Autodesk Fusion 360 part; units mm, degrees
(part 2 of 3)
  line L328 (-114.4464, -236.9799) -> (-114.4464, -230.9799)
  line L329 (-114.4464, -230.9799) -> (-108.4464, -230.9799)
  line L330 (-108.4464, -230.9799) -> (-108.4464, -236.9799)
  line L331 (-108.4464, -236.9799) -> (-114.4464, -236.9799)
  line L332 (53.6667, -182.5) -> (47.6667, -182.5)
  line L333 (47.6667, -182.5) -> (47.6667, -176.5)
  line L334 (47.6667, -176.5) -> (53.6667, -176.5)
  line L335 (53.6667, -176.5) -> (53.6667, -182.5)
  line L336 (61.3333, -182.5) -> (55.3333, -182.5)
  line L337 (55.3333, -182.5) -> (55.3333, -176.5)
  line L338 (55.3333, -176.5) -> (61.3333, -176.5)
  line L339 (61.3333, -176.5) -> (61.3333, -182.5)
  line L340 (69, -182.5) -> (63, -182.5)
  line L341 (63, -182.5) -> (63, -176.5)
  line L342 (63, -176.5) -> (69, -176.5)
  line L343 (69, -176.5) -> (69, -182.5)
  line L344 (76.6667, -182.5) -> (70.6667, -182.5)
  line L345 (70.6667, -182.5) -> (70.6667, -176.5)
  line L346 (70.6667, -176.5) -> (76.6667, -176.5)
  line L347 (76.6667, -176.5) -> (76.6667, -182.5)
  line L348 (84.3333, -182.5) -> (78.3333, -182.5)
  line L349 (78.3333, -182.5) -> (78.3333, -176.5)
  line L350 (78.3333, -176.5) -> (84.3333, -176.5)
  line L351 (84.3333, -176.5) -> (84.3333, -182.5)
  line L352 (92, -182.5) -> (86, -182.5)
  line L353 (86, -182.5) -> (86, -176.5)
  line L354 (86, -176.5) -> (92, -176.5)
  line L355 (92, -176.5) -> (92, -182.5)
  line L356 (99.6667, -182.5) -> (93.6667, -182.5)
  line L357 (93.6667, -182.5) -> (93.6667, -176.5)
  line L358 (93.6667, -176.5) -> (99.6667, -176.5)
  line L359 (99.6667, -176.5) -> (99.6667, -182.5)
  line L360 (107.3333, -182.5) -> (101.3333, -182.5)
  line L361 (101.3333, -182.5) -> (101.3333, -176.5)
  line L362 (101.3333, -176.5) -> (107.3333, -176.5)
  line L363 (107.3333, -176.5) -> (107.3333, -182.5)
  line L364 (53.6667, -190.3571) -> (47.6667, -190.3571)
  line L365 (47.6667, -190.3571) -> (47.6667, -184.3571)
  line L366 (47.6667, -184.3571) -> (53.6667, -184.3571)
  line L367 (53.6667, -184.3571) -> (53.6667, -190.3571)
  line L368 (61.3333, -190.3571) -> (55.3333, -190.3571)
  line L369 (55.3333, -190.3571) -> (55.3333, -184.3571)
  line L370 (55.3333, -184.3571) -> (61.3333, -184.3571)
  line L371 (61.3333, -184.3571) -> (61.3333, -190.3571)
  line L372 (69, -190.3571) -> (63, -190.3571)
  line L373 (63, -190.3571) -> (63, -184.3571)
  line L374 (63, -184.3571) -> (69, -184.3571)
  line L375 (69, -184.3571) -> (69, -190.3571)
  line L376 (76.6667, -190.3571) -> (70.6667, -190.3571)
  line L377 (70.6667, -190.3571) -> (70.6667, -184.3571)
  line L378 (70.6667, -184.3571) -> (76.6667, -184.3571)
  line L379 (76.6667, -184.3571) -> (76.6667, -190.3571)
  line L380 (84.3333, -190.3571) -> (78.3333, -190.3571)
  line L381 (78.3333, -190.3571) -> (78.3333, -184.3571)
  line L382 (78.3333, -184.3571) -> (84.3333, -184.3571)
  line L383 (84.3333, -184.3571) -> (84.3333, -190.3571)
  line L384 (92, -190.3571) -> (86, -190.3571)
  line L385 (86, -190.3571) -> (86, -184.3571)
  line L386 (86, -184.3571) -> (92, -184.3571)
  line L387 (92, -184.3571) -> (92, -190.3571)
  line L388 (99.6667, -190.3571) -> (93.6667, -190.3571)
  line L389 (93.6667, -190.3571) -> (93.6667, -184.3571)
  line L390 (93.6667, -184.3571) -> (99.6667, -184.3571)
  line L391 (99.6667, -184.3571) -> (99.6667, -190.3571)
  line L392 (107.3333, -190.3571) -> (101.3333, -190.3571)
  line L393 (101.3333, -190.3571) -> (101.3333, -184.3571)
  line L394 (101.3333, -184.3571) -> (107.3333, -184.3571)
  line L395 (107.3333, -184.3571) -> (107.3333, -190.3571)
  line L396 (53.6667, -198.2143) -> (47.6667, -198.2143)
  line L397 (47.6667, -198.2143) -> (47.6667, -192.2143)
  line L398 (47.6667, -192.2143) -> (53.6667, -192.2143)
  line L399 (53.6667, -192.2143) -> (53.6667, -198.2143)
  line L400 (61.3333, -198.2143) -> (55.3333, -198.2143)
  line L401 (55.3333, -198.2143) -> (55.3333, -192.2143)
  line L402 (55.3333, -192.2143) -> (61.3333, -192.2143)
  line L403 (61.3333, -192.2143) -> (61.3333, -198.2143)
  line L404 (69, -198.2143) -> (63, -198.2143)
  line L405 (63, -198.2143) -> (63, -192.2143)
  line L406 (63, -192.2143) -> (69, -192.2143)
  line L407 (69, -192.2143) -> (69, -198.2143)
  line L408 (76.6667, -198.2143) -> (70.6667, -198.2143)
  line L409 (70.6667, -198.2143) -> (70.6667, -192.2143)
  line L410 (70.6667, -192.2143) -> (76.6667, -192.2143)
  line L411 (76.6667, -192.2143) -> (76.6667, -198.2143)
  line L412 (84.3333, -198.2143) -> (78.3333, -198.2143)
  line L413 (78.3333, -198.2143) -> (78.3333, -192.2143)
  line L414 (78.3333, -192.2143) -> (84.3333, -192.2143)
  line L415 (84.3333, -192.2143) -> (84.3333, -198.2143)
  line L416 (92, -198.2143) -> (86, -198.2143)
  line L417 (86, -198.2143) -> (86, -192.2143)
  line L418 (86, -192.2143) -> (92, -192.2143)
  line L419 (92, -192.2143) -> (92, -198.2143)
  line L420 (99.6667, -198.2143) -> (93.6667, -198.2143)
  line L421 (93.6667, -198.2143) -> (93.6667, -192.2143)
  line L422 (93.6667, -192.2143) -> (99.6667, -192.2143)
  line L423 (99.6667, -192.2143) -> (99.6667, -198.2143)
  line L424 (107.3333, -198.2143) -> (101.3333, -198.2143)
  line L425 (101.3333, -198.2143) -> (101.3333, -192.2143)
  line L426 (101.3333, -192.2143) -> (107.3333, -192.2143)
  line L427 (107.3333, -192.2143) -> (107.3333, -198.2143)
  line L428 (53.6667, -206.0714) -> (47.6667, -206.0714)
  line L429 (47.6667, -206.0714) -> (47.6667, -200.0714)
  line L430 (47.6667, -200.0714) -> (53.6667, -200.0714)
  line L431 (53.6667, -200.0714) -> (53.6667, -206.0714)
  line L432 (61.3333, -206.0714) -> (55.3333, -206.0714)
  line L433 (55.3333, -206.0714) -> (55.3333, -200.0714)
  line L434 (55.3333, -200.0714) -> (61.3333, -200.0714)
  line L435 (61.3333, -200.0714) -> (61.3333, -206.0714)
  line L436 (69, -206.0714) -> (63, -206.0714)
  line L437 (63, -206.0714) -> (63, -200.0714)
  line L438 (63, -200.0714) -> (69, -200.0714)
  line L439 (69, -200.0714) -> (69, -206.0714)
  line L440 (76.6667, -206.0714) -> (70.6667, -206.0714)
  line L441 (70.6667, -206.0714) -> (70.6667, -200.0714)
  line L442 (70.6667, -200.0714) -> (76.6667, -200.0714)
  line L443 (76.6667, -200.0714) -> (76.6667, -206.0714)
  line L444 (84.3333, -206.0714) -> (78.3333, -206.0714)
  line L445 (78.3333, -206.0714) -> (78.3333, -200.0714)
  line L446 (78.3333, -200.0714) -> (84.3333, -200.0714)
  line L447 (84.3333, -200.0714) -> (84.3333, -206.0714)
  line L448 (92, -206.0714) -> (86, -206.0714)
  line L449 (86, -206.0714) -> (86, -200.0714)
  line L450 (86, -200.0714) -> (92, -200.0714)
  line L451 (92, -200.0714) -> (92, -206.0714)
  line L452 (99.6667, -206.0714) -> (93.6667, -206.0714)
  line L453 (93.6667, -206.0714) -> (93.6667, -200.0714)
  line L454 (93.6667, -200.0714) -> (99.6667, -200.0714)
  line L455 (99.6667, -200.0714) -> (99.6667, -206.0714)
  line L456 (107.3333, -206.0714) -> (101.3333, -206.0714)
  line L457 (101.3333, -206.0714) -> (101.3333, -200.0714)
  line L458 (101.3333, -200.0714) -> (107.3333, -200.0714)
  line L459 (107.3333, -200.0714) -> (107.3333, -206.0714)
  line L460 (53.6667, -213.9286) -> (47.6667, -213.9286)
  line L461 (47.6667, -213.9286) -> (47.6667, -207.9286)
  line L462 (47.6667, -207.9286) -> (53.6667, -207.9286)
  line L463 (53.6667, -207.9286) -> (53.6667, -213.9286)
  line L464 (61.3333, -213.9286) -> (55.3333, -213.9286)
  line L465 (55.3333, -213.9286) -> (55.3333, -207.9286)
  line L466 (55.3333, -207.9286) -> (61.3333, -207.9286)
  line L467 (61.3333, -207.9286) -> (61.3333, -213.9286)
  line L468 (69, -213.9286) -> (63, -213.9286)
  line L469 (63, -213.9286) -> (63, -207.9286)
  line L470 (63, -207.9286) -> (69, -207.9286)
  line L471 (69, -207.9286) -> (69, -213.9286)
  line L472 (76.6667, -213.9286) -> (70.6667, -213.9286)
  line L473 (70.6667, -213.9286) -> (70.6667, -207.9286)
  line L474 (70.6667, -207.9286) -> (76.6667, -207.9286)
  line L475 (76.6667, -207.9286) -> (76.6667, -213.9286)
  line L476 (84.3333, -213.9286) -> (78.3333, -213.9286)
  line L477 (78.3333, -213.9286) -> (78.3333, -207.9286)
  line L478 (78.3333, -207.9286) -> (84.3333, -207.9286)
  line L479 (84.3333, -207.9286) -> (84.3333, -213.9286)
  line L480 (92, -213.9286) -> (86, -213.9286)
  line L481 (86, -213.9286) -> (86, -207.9286)
  line L482 (86, -207.9286) -> (92, -207.9286)
  line L483 (92, -207.9286) -> (92, -213.9286)
  line L484 (99.6667, -213.9286) -> (93.6667, -213.9286)
  line L485 (93.6667, -213.9286) -> (93.6667, -207.9286)
  line L486 (93.6667, -207.9286) -> (99.6667, -207.9286)
  line L487 (99.6667, -207.9286) -> (99.6667, -213.9286)
  line L488 (107.3333, -213.9286) -> (101.3333, -213.9286)
  line L489 (101.3333, -213.9286) -> (101.3333, -207.9286)
  line L490 (101.3333, -207.9286) -> (107.3333, -207.9286)
  line L491 (107.3333, -207.9286) -> (107.3333, -213.9286)
  line L492 (53.6667, -221.7857) -> (47.6667, -221.7857)
  line L493 (47.6667, -221.7857) -> (47.6667, -215.7857)
  line L494 (47.6667, -215.7857) -> (53.6667, -215.7857)
  line L495 (53.6667, -215.7857) -> (53.6667, -221.7857)
  line L496 (61.3333, -221.7857) -> (55.3333, -221.7857)
  line L497 (55.3333, -221.7857) -> (55.3333, -215.7857)
  line L498 (55.3333, -215.7857) -> (61.3333, -215.7857)
  line L499 (61.3333, -215.7857) -> (61.3333, -221.7857)
  line L500 (69, -221.7857) -> (63, -221.7857)
  line L501 (63, -221.7857) -> (63, -215.7857)
  line L502 (63, -215.7857) -> (69, -215.7857)
  line L503 (69, -215.7857) -> (69, -221.7857)
  line L504 (76.6667, -221.7857) -> (70.6667, -221.7857)
  line L505 (70.6667, -221.7857) -> (70.6667, -215.7857)
  line L506 (70.6667, -215.7857) -> (76.6667, -215.7857)
  line L507 (76.6667, -215.7857) -> (76.6667, -221.7857)
  line L508 (84.3333, -221.7857) -> (78.3333, -221.7857)
  line L509 (78.3333, -221.7857) -> (78.3333, -215.7857)
  line L510 (78.3333, -215.7857) -> (84.3333, -215.7857)
  line L511 (84.3333, -215.7857) -> (84.3333, -221.7857)
  line L512 (92, -221.7857) -> (86, -221.7857)
  line L513 (86, -221.7857) -> (86, -215.7857)
  line L514 (86, -215.7857) -> (92, -215.7857)
  line L515 (92, -215.7857) -> (92, -221.7857)
  line L516 (99.6667, -221.7857) -> (93.6667, -221.7857)
  line L517 (93.6667, -221.7857) -> (93.6667, -215.7857)
  line L518 (93.6667, -215.7857) -> (99.6667, -215.7857)
  line L519 (99.6667, -215.7857) -> (99.6667, -221.7857)
  line L520 (107.3333, -221.7857) -> (101.3333, -221.7857)
  line L521 (101.3333, -221.7857) -> (101.3333, -215.7857)
  line L522 (101.3333, -215.7857) -> (107.3333, -215.7857)
  line L523 (107.3333, -215.7857) -> (107.3333, -221.7857)
  line L524 (53.6667, -229.6429) -> (47.6667, -229.6429)
  line L525 (47.6667, -229.6429) -> (47.6667, -223.6429)
  line L526 (47.6667, -223.6429) -> (53.6667, -223.6429)
  line L527 (53.6667, -223.6429) -> (53.6667, -229.6429)
  line L528 (61.3333, -229.6429) -> (55.3333, -229.6429)
  line L529 (55.3333, -229.6429) -> (55.3333, -223.6429)
  line L530 (55.3333, -223.6429) -> (61.3333, -223.6429)
  line L531 (61.3333, -223.6429) -> (61.3333, -229.6429)
  line L532 (69, -229.6429) -> (63, -229.6429)
  line L533 (63, -229.6429) -> (63, -223.6429)
  line L534 (63, -223.6429) -> (69, -223.6429)
  line L535 (69, -223.6429) -> (69, -229.6429)
  line L536 (76.6667, -229.6429) -> (70.6667, -229.6429)
  line L537 (70.6667, -229.6429) -> (70.6667, -223.6429)
  line L538 (70.6667, -223.6429) -> (76.6667, -223.6429)
  line L539 (76.6667, -223.6429) -> (76.6667, -229.6429)
  line L540 (84.3333, -229.6429) -> (78.3333, -229.6429)
  line L541 (78.3333, -229.6429) -> (78.3333, -223.6429)
  line L542 (78.3333, -223.6429) -> (84.3333, -223.6429)
  line L543 (84.3333, -223.6429) -> (84.3333, -229.6429)
  line L544 (92, -229.6429) -> (86, -229.6429)
  line L545 (86, -229.6429) -> (86, -223.6429)
  line L546 (86, -223.6429) -> (92, -223.6429)
  line L547 (92, -223.6429) -> (92, -229.6429)
  line L548 (99.6667, -229.6429) -> (93.6667, -229.6429)
  line L549 (93.6667, -229.6429) -> (93.6667, -223.6429)
  line L550 (93.6667, -223.6429) -> (99.6667, -223.6429)
  line L551 (99.6667, -223.6429) -> (99.6667, -229.6429)
  line L552 (107.3333, -229.6429) -> (101.3333, -229.6429)
  line L553 (101.3333, -229.6429) -> (101.3333, -223.6429)
  line L554 (101.3333, -223.6429) -> (107.3333, -223.6429)
  line L555 (107.3333, -223.6429) -> (107.3333, -229.6429)
  line L556 (53.6667, -237.5) -> (47.6667, -237.5)
  line L557 (47.6667, -237.5) -> (47.6667, -231.5)
  line L558 (47.6667, -231.5) -> (53.6667, -231.5)
  line L559 (53.6667, -231.5) -> (53.6667, -237.5)
  line L560 (61.3333, -237.5) -> (55.3333, -237.5)
  line L561 (55.3333, -237.5) -> (55.3333, -231.5)
  line L562 (55.3333, -231.5) -> (61.3333, -231.5)
  line L563 (61.3333, -231.5) -> (61.3333, -237.5)
  line L564 (69, -237.5) -> (63, -237.5)
  line L565 (63, -237.5) -> (63, -231.5)
  line L566 (63, -231.5) -> (69, -231.5)
  line L567 (69, -231.5) -> (69, -237.5)
  line L568 (76.6667, -237.5) -> (70.6667, -237.5)
  line L569 (70.6667, -237.5) -> (70.6667, -231.5)
  line L570 (70.6667, -231.5) -> (76.6667, -231.5)
  line L571 (76.6667, -231.5) -> (76.6667, -237.5)
  line L572 (84.3333, -237.5) -> (78.3333, -237.5)
  line L573 (78.3333, -237.5) -> (78.3333, -231.5)
  line L574 (78.3333, -231.5) -> (84.3333, -231.5)
  line L575 (84.3333, -231.5) -> (84.3333, -237.5)
  line L576 (92, -237.5) -> (86, -237.5)
  line L577 (86, -237.5) -> (86, -231.5)
  line L578 (86, -231.5) -> (92, -231.5)
  line L579 (92, -231.5) -> (92, -237.5)
  line L580 (99.6667, -237.5) -> (93.6667, -237.5)
  line L581 (93.6667, -237.5) -> (93.6667, -231.5)
  line L582 (93.6667, -231.5) -> (99.6667, -231.5)
  line L583 (99.6667, -231.5) -> (99.6667, -237.5)
  line L584 (101.3333, -231.5) -> (107.3333, -231.5)
  line L585 (107.3333, -231.5) -> (107.3333, -237.5)
  line L586 (107.3333, -237.5) -> (101.3333, -237.5)
  line L587 (101.3333, -237.5) -> (101.3333, -231.5)
  line L588 (156, -177) -> (156, -160)
  line L589 (156, -160) -> (143.1111, -160)
  line L590 (143.1111, -160) -> (143.1111, -155)
  line L591 (143.1111, -155) -> (125.2222, -155)
  line L592 (125.2222, -155) -> (125.2222, -160)
  line L593 (125.2222, -160) -> (107.3333, -160)
  line L594 (107.3333, -160) -> (107.3333, -155)
  line L595 (107.3333, -155) -> (89.4444, -155)
  line L596 (89.4444, -155) -> (89.4444, -160)
  line L597 (89.4444, -160) -> (71.5556, -160)
  line L598 (71.5556, -160) -> (71.5556, -155)
  line L599 (71.5556, -155) -> (53.6667, -155)
  line L600 (53.6667, -155) -> (53.6667, -160)
  line L601 (53.6667, -160) -> (35.7778, -160)
  line L602 (35.7778, -160) -> (35.7778, -155)
  line L603 (35.7778, -155) -> (17.8889, -155)
  line L604 (17.8889, -155) -> (17.8889, -160)
  line L605 (17.8889, -160) -> (5, -160)
  line L606 (5, -160) -> (5, -177)
  line L607 (5, -177) -> (0, -177)
  line L608 (0, -177) -> (0, -199)
  line L609 (0, -199) -> (5, -199)
  line L610 (5, -199) -> (5, -221)
  line L611 (5, -221) -> (0, -221)
  line L612 (0, -221) -> (0, -243)
  line L613 (0, -243) -> (5, -243)
  line L614 (5, -243) -> (5, -265)
  line L615 (5, -265) -> (156, -265)
  line L616 (156, -265) -> (156, -243)
  line L617 (156, -243) -> (161, -243)
  line L618 (161, -243) -> (161, -221)
  line L619 (161, -221) -> (156, -221)
  line L620 (156, -221) -> (156, -199)
  line L621 (156, -199) -> (161, -199)
  line L622 (161, -199) -> (161, -177)
  line L623 (161, -177) -> (156, -177)
  line L624 (264.348, -187.6487) -> (264.348, -172.6487)
  line L625 (264.348, -172.6487) -> (270.348, -172.6487)
  line L626 (270.348, -172.6487) -> (270.348, -187.6487)
  line L627 (270.348, -187.6487) -> (264.348, -187.6487)
  line L628 (256.0147, -187.6487) -> (256.0147, -172.6487)
  line L629 (256.0147, -172.6487) -> (262.0147, -172.6487)
  line L630 (262.0147, -172.6487) -> (262.0147, -187.6487)
  line L631 (262.0147, -187.6487) -> (256.0147, -187.6487)
  line L632 (247.6814, -187.6487) -> (247.6814, -172.6487)
  line L633 (247.6814, -172.6487) -> (253.6814, -172.6487)
  line L634 (253.6814, -172.6487) -> (253.6814, -187.6487)
  line L635 (253.6814, -187.6487) -> (247.6814, -187.6487)
  line L636 (239.348, -187.6487) -> (239.348, -172.6487)
  line L637 (239.348, -172.6487) -> (245.348, -172.6487)
  line L638 (245.348, -172.6487) -> (245.348, -187.6487)
  line L639 (245.348, -187.6487) -> (239.348, -187.6487)
  line L640 (231.0147, -187.6487) -> (231.0147, -172.6487)
  line L641 (231.0147, -172.6487) -> (237.0147, -172.6487)
  line L642 (237.0147, -172.6487) -> (237.0147, -187.6487)
  line L643 (237.0147, -187.6487) -> (231.0147, -187.6487)
  line L644 (222.6814, -187.6487) -> (222.6814, -172.6487)
  line L645 (222.6814, -172.6487) -> (228.6814, -172.6487)
  line L646 (228.6814, -172.6487) -> (228.6814, -187.6487)
  line L647 (228.6814, -187.6487) -> (222.6814, -187.6487)
  line L648 (214.348, -187.6487) -> (214.348, -172.6487)
  line L649 (214.348, -172.6487) -> (220.348, -172.6487)
  line L650 (220.348, -172.6487) -> (220.348, -187.6487)
  line L651 (220.348, -187.6487) -> (214.348, -187.6487)
  line L652 (206.0147, -187.6487) -> (206.0147, -172.6487)
  line L653 (206.0147, -172.6487) -> (212.0147, -172.6487)
  line L654 (212.0147, -172.6487) -> (212.0147, -187.6487)
  line L655 (212.0147, -187.6487) -> (206.0147, -187.6487)
  line L656 (197.6814, -187.6487) -> (197.6814, -172.6487)
  line L657 (197.6814, -172.6487) -> (203.6814, -172.6487)
  line L658 (203.6814, -172.6487) -> (203.6814, -187.6487)
  line L659 (203.6814, -187.6487) -> (197.6814, -187.6487)
  line L660 (189.348, -187.6487) -> (189.348, -172.6487)
  line L661 (189.348, -172.6487) -> (195.348, -172.6487)
  line L662 (195.348, -172.6487) -> (195.348, -187.6487)
  line L663 (195.348, -187.6487) -> (189.348, -187.6487)
  line L664 (309.348, -176.3154) -> (314.348, -176.3154)
  line L665 (314.348, -176.3154) -> (314.348, -159.3154)
  line L666 (314.348, -159.3154) -> (300.7117, -159.3154)
  line L667 (300.7117, -159.3154) -> (300.7117, -154.3154)
  line L668 (300.7117, -154.3154) -> (287.0753, -154.3154)
  line L669 (287.0753, -154.3154) -> (287.0753, -159.3154)
  line L670 (287.0753, -159.3154) -> (273.4389, -159.3154)
  line L671 (273.4389, -159.3154) -> (273.4389, -154.3154)
  line L672 (273.4389, -154.3154) -> (259.8026, -154.3154)
  line L673 (259.8026, -154.3154) -> (259.8026, -159.3154)
  line L674 (259.8026, -159.3154) -> (246.1662, -159.3154)
  line L675 (246.1662, -159.3154) -> (246.1662, -154.3154)
  line L676 (246.1662, -154.3154) -> (232.5298, -154.3154)
  line L677 (232.5298, -154.3154) -> (232.5298, -159.3154)
  line L678 (232.5298, -159.3154) -> (218.8935, -159.3154)
  line L679 (218.8935, -159.3154) -> (218.8935, -154.3154)
  line L680 (218.8935, -154.3154) -> (205.2571, -154.3154)
  line L681 (205.2571, -154.3154) -> (205.2571, -159.3154)
  line L682 (205.2571, -159.3154) -> (191.6208, -159.3154)
  line L683 (191.6208, -159.3154) -> (191.6208, -154.3154)
  line L684 (191.6208, -154.3154) -> (177.9844, -154.3154)
  line L685 (177.9844, -154.3154) -> (177.9844, -159.3154)
  line L686 (177.9844, -159.3154) -> (164.348, -159.3154)
  line L687 (164.348, -159.3154) -> (164.348, -176.3154)
  line L688 (164.348, -176.3154) -> (169.348, -176.3154)
  line L689 (169.348, -176.3154) -> (169.348, -198.3154)
  line L690 (169.348, -198.3154) -> (164.348, -198.3154)
  line L691 (164.348, -198.3154) -> (164.348, -220.3154)
  line L692 (164.348, -220.3154) -> (169.348, -220.3154)
  line L693 (169.348, -220.3154) -> (169.348, -242.3154)
  line L694 (169.348, -242.3154) -> (164.348, -242.3154)
  line L695 (164.348, -242.3154) -> (164.348, -264.3154)
  line L696 (164.348, -264.3154) -> (314.348, -264.3154)
  line L697 (314.348, -264.3154) -> (314.348, -242.3154)
  line L698 (314.348, -242.3154) -> (309.348, -242.3154)
  line L699 (309.348, -242.3154) -> (309.348, -220.3154)
  line L700 (309.348, -220.3154) -> (314.348, -220.3154)
  line L701 (314.348, -220.3154) -> (314.348, -198.3154)
  line L702 (314.348, -198.3154) -> (309.348, -198.3154)
  line L703 (309.348, -198.3154) -> (309.348, -176.3154)
  line L704 (338.3812, -119.0374) -> (338.3812, -114.0374)
  line L705 (338.3812, -114.0374) -> (320.4923, -114.0374)
  line L706 (320.4923, -114.0374) -> (320.4923, -127.6738)
  line L707 (320.4923, -127.6738) -> (325.4923, -127.6738)
  line L708 (325.4923, -127.6738) -> (325.4923, -141.3101)
  line L709 (325.4923, -141.3101) -> (320.4923, -141.3101)
  line L710 (320.4923, -141.3101) -> (320.4923, -154.9465)
  line L711 (320.4923, -154.9465) -> (325.4923, -154.9465)
  line L712 (325.4923, -154.9465) -> (325.4923, -168.5829)
  line L713 (325.4923, -168.5829) -> (320.4923, -168.5829)
  line L714 (320.4923, -168.5829) -> (320.4923, -182.2192)
  line L715 (320.4923, -182.2192) -> (325.4923, -182.2192)
  line L716 (325.4923, -182.2192) -> (325.4923, -195.8556)
  line L717 (325.4923, -195.8556) -> (320.4923, -195.8556)
  line L718 (320.4923, -195.8556) -> (320.4923, -209.492)
  line L719 (320.4923, -209.492) -> (325.4923, -209.492)
  line L720 (325.4923, -209.492) -> (325.4923, -223.1283)
  line L721 (325.4923, -223.1283) -> (320.4923, -223.1283)
  line L722 (320.4923, -223.1283) -> (320.4923, -236.7647)
  line L723 (320.4923, -236.7647) -> (325.4923, -236.7647)
  line L724 (325.4923, -236.7647) -> (325.4923, -250.401)
  line L725 (325.4923, -250.401) -> (320.4923, -250.401)
  line L726 (320.4923, -250.401) -> (320.4923, -264.0374)
  line L727 (320.4923, -264.0374) -> (338.3812, -264.0374)
  line L728 (338.3812, -264.0374) -> (338.3812, -259.0374)
  line L729 (338.3812, -259.0374) -> (356.2701, -259.0374)
  line L730 (356.2701, -259.0374) -> (356.2701, -264.0374)
  line L731 (356.2701, -264.0374) -> (374.159, -264.0374)
  line L732 (374.159, -264.0374) -> (374.159, -259.0374)
  line L733 (374.159, -259.0374) -> (392.0478, -259.0374)
  line L734 (392.0478, -259.0374) -> (392.0478, -264.0374)
  line L735 (392.0478, -264.0374) -> (409.9367, -264.0374)
  line L736 (409.9367, -264.0374) -> (409.9367, -259.0374)
  line L737 (409.9367, -259.0374) -> (427.8256, -259.0374)
  line L738 (427.8256, -259.0374) -> (427.8256, -264.0374)
  line L739 (427.8256, -264.0374) -> (445.7145, -264.0374)
  line L740 (445.7145, -264.0374) -> (445.7145, -259.0374)
  line L741 (445.7145, -259.0374) -> (463.6034, -259.0374)
  line L742 (463.6034, -259.0374) -> (463.6034, -264.0374)
  line L743 (463.6034, -264.0374) -> (481.4923, -264.0374)
  line L744 (481.4923, -264.0374) -> (481.4923, -250.401)
  line L745 (481.4923, -250.401) -> (476.4923, -250.401)
  line L746 (476.4923, -250.401) -> (476.4923, -236.7647)
  line L747 (476.4923, -236.7647) -> (481.4923, -236.7647)
  line L748 (481.4923, -236.7647) -> (481.4923, -223.1283)
  line L749 (481.4923, -223.1283) -> (476.4923, -223.1283)
  line L750 (476.4923, -223.1283) -> (476.4923, -209.492)
  line L751 (476.4923, -209.492) -> (481.4923, -209.492)
  line L752 (481.4923, -209.492) -> (481.4923, -195.8556)
  line L753 (481.4923, -195.8556) -> (476.4923, -195.8556)
  line L754 (476.4923, -195.8556) -> (476.4923, -182.2192)
  line L755 (476.4923, -182.2192) -> (481.4923, -182.2192)
  line L756 (481.4923, -182.2192) -> (481.4923, -168.5829)
  line L757 (481.4923, -168.5829) -> (476.4923, -168.5829)
  line L758 (476.4923, -168.5829) -> (476.4923, -154.9465)
  line L759 (476.4923, -154.9465) -> (481.4923, -154.9465)
  line L760 (481.4923, -154.9465) -> (481.4923, -141.3101)
  line L761 (481.4923, -141.3101) -> (476.4923, -141.3101)
  line L762 (476.4923, -141.3101) -> (476.4923, -127.6738)
  line L763 (476.4923, -127.6738) -> (481.4923, -127.6738)
  line L764 (481.4923, -127.6738) -> (481.4923, -114.0374)
  line L765 (481.4923, -114.0374) -> (463.6034, -114.0374)
  line L766 (463.6034, -114.0374) -> (463.6034, -119.0374)
  line L767 (463.6034, -119.0374) -> (445.7145, -119.0374)
  line L768 (445.7145, -119.0374) -> (445.7145, -114.0374)
  line L769 (445.7145, -114.0374) -> (427.8256, -114.0374)
  line L770 (427.8256, -114.0374) -> (427.8256, -119.0374)
  line L771 (427.8256, -119.0374) -> (409.9367, -119.0374)
  line L772 (409.9367, -119.0374) -> (409.9367, -114.0374)
  line L773 (409.9367, -114.0374) -> (392.0478, -114.0374)
  line L774 (392.0478, -114.0374) -> (392.0478, -119.0374)
  line L775 (392.0478, -119.0374) -> (374.159, -119.0374)
  line L776 (374.159, -119.0374) -> (374.159, -114.0374)
  line L777 (374.159, -114.0374) -> (356.2701, -114.0374)
  line L778 (356.2701, -114.0374) -> (356.2701, -119.0374)
  line L779 (356.2701, -119.0374) -> (338.3812, -119.0374)
  line L780 (-317.0163, -146.5816) -> (-262.0163, -146.5816)
  arc A4 (-262.0163, -146.5816) -> (-317.0163, -146.5816) centre (-289.5163, -176.6927) ccw
  line L781 (-251.0163, -146.5816) -> (-196.0163, -146.5816)
  arc A5 (-196.0163, -146.5816) -> (-251.0163, -146.5816) centre (-223.5163, -176.6927) ccw
  line L782 (-185.0163, -146.5816) -> (-130.0163, -146.5816)
  arc A6 (-130.0163, -146.5816) -> (-185.0163, -146.5816) centre (-157.5163, -176.6927) ccw
  line L783 (-119.0163, -146.5816) -> (-64.0163, -146.5816)
  arc A7 (-64.0163, -146.5816) -> (-119.0163, -146.5816) centre (-91.5163, -176.6927) ccw
  line L784 (-53.0163, -146.5816) -> (1.9837, -146.5816)
  arc A8 (1.9837, -146.5816) -> (-53.0163, -146.5816) centre (-25.5163, -176.6927) ccw
  line L785 (12.9837, -146.5816) -> (67.9837, -146.5816)
  arc A9 (67.9837, -146.5816) -> (12.9837, -146.5816) centre (40.4837, -176.6927) ccw
  line L786 (-453.7776, -187.2012) -> (-343.7776, -187.2012)
  line L787 (-343.7776, -187.2012) -> (-343.7776, -217.2012)
  line L788 (-343.7776, -217.2012) -> (-453.7776, -217.2012)
  line L789 (-453.7776, -217.2012) -> (-453.7776, -187.2012)
  line L790 (-463.9983, -178.5266) -> (-333.9983, -178.5266)
  line L791 (-333.9983, -178.5266) -> (-333.9983, -263.5266)
  line L792 (-333.9983, -263.5266) -> (-463.9983, -263.5266)
  line L793 (-463.9983, -263.5266) -> (-463.9983, -178.5266)
  line L794 (195, -195) -> (220, -195)
  line L795 (220, -195) -> (220, -205)
  line L796 (220, -205) -> (195, -205)
  line L797 (195, -205) -> (195, -195)
  line L798 (235, -195) -> (260, -195)
  line L799 (260, -195) -> (260, -205)
  line L800 (260, -205) -> (235, -205)
  line L801 (235, -205) -> (235, -195)
  line L802 (198, -196) -> (217, -196)
  line L803 (217, -196) -> (217, -201)
  line L804 (217, -201) -> (212, -202)
  line L805 (212, -202) -> (203, -202)
  line L806 (203, -202) -> (198, -201)
  line L807 (198, -201) -> (198, -196)
  line L808 (238, -196) -> (238, -202)
  line L809 (238, -202) -> (240, -204)
  line L810 (240, -204) -> (255, -204)
  line L811 (255, -204) -> (257, -202)
  line L812 (257, -202) -> (257, -196)
  line L813 (257, -196) -> (238, -196)
  line L814 (-459.0497, -136.1366) -> (-338.2997, -136.1366)
  line L815 (-338.2997, -136.1366) -> (-338.2997, -172.8032)
  line L816 (-338.2997, -172.8032) -> (-459.0497, -172.8032)
  line L817 (-459.0497, -172.8032) -> (-459.0497, -136.1366)
  line L818 (-445.2487, -136.1366) -> (-442.2487, -136.1366)
  line L819 (-442.2487, -172.8032) -> (-445.2487, -172.8032)
  line L820 (-445.2487, -172.8032) -> (-445.2487, -163.6366)
  line L821 (-445.2487, -136.1366) -> (-445.2487, -145.3032)
  line L822 (-442.2487, -142.0103) -> (-442.2487, -151.177)
  line L823 (-442.2487, -165.4723) -> (-442.2487, -156.3057)
  line L824 (-445.2487, -154.4699) -> (-445.2487, -149.8866)
  line L825 (-445.2487, -154.4699) -> (-445.2487, -159.0532)
  line L826 (-440.3462, -172.8032) -> (-440.3462, -163.6366)
  line L827 (-437.3462, -165.4723) -> (-437.3462, -156.3057)
  line L828 (-440.3462, -154.4699) -> (-440.3462, -159.0532)
  line L829 (-440.3462, -154.4699) -> (-440.3462, -149.8866)
  line L830 (-437.3462, -142.0103) -> (-437.3462, -151.177)
  line L831 (-440.3462, -136.1366) -> (-440.3462, -145.3032)
  line L832 (-435.4437, -172.8032) -> (-435.4437, -163.6366)
  line L833 (-432.4437, -165.4723) -> (-432.4437, -156.3057)
  line L834 (-435.4437, -154.4699) -> (-435.4437, -159.0532)
  line L835 (-435.4437, -154.4699) -> (-435.4437, -149.8866)
  line L836 (-432.4437, -142.0103) -> (-432.4437, -151.177)
  line L837 (-435.4437, -136.1366) -> (-435.4437, -145.3032)
  line L838 (-430.5412, -172.8032) -> (-430.5412, -163.6366)
  line L839 (-427.5412, -165.4723) -> (-427.5412, -156.3057)
  line L840 (-430.5412, -154.4699) -> (-430.5412, -159.0532)
  line L841 (-430.5412, -154.4699) -> (-430.5412, -149.8866)
  line L842 (-427.5412, -142.0103) -> (-427.5412, -151.177)
  line L843 (-430.5412, -136.1366) -> (-430.5412, -145.3032)
  line L844 (-425.6386, -172.8032) -> (-425.6386, -163.6366)
  line L845 (-422.6386, -165.4723) -> (-422.6386, -156.3057)
  line L846 (-425.6386, -154.4699) -> (-425.6386, -159.0532)
  line L847 (-425.6386, -154.4699) -> (-425.6386, -149.8866)
  line L848 (-422.6386, -142.0103) -> (-422.6386, -151.177)
  line L849 (-425.6386, -136.1366) -> (-425.6386, -145.3032)
  line L850 (-420.7361, -172.8032) -> (-420.7361, -163.6366)
  line L851 (-417.7361, -165.4723) -> (-417.7361, -156.3057)
  line L852 (-420.7361, -154.4699) -> (-420.7361, -159.0532)
  line L853 (-420.7361, -154.4699) -> (-420.7361, -149.8866)
  line L854 (-417.7361, -142.0103) -> (-417.7361, -151.177)
  line L855 (-420.7361, -136.1366) -> (-420.7361, -145.3032)
  line L856 (-415.8336, -172.8032) -> (-415.8336, -163.6366)
  line L857 (-412.8336, -165.4723) -> (-412.8336, -156.3057)
  line L858 (-415.8336, -154.4699) -> (-415.8336, -159.0532)
  line L859 (-415.8336, -154.4699) -> (-415.8336, -149.8866)
  line L860 (-412.8336, -142.0103) -> (-412.8336, -151.177)
  line L861 (-415.8336, -136.1366) -> (-415.8336, -145.3032)
  line L862 (-410.9311, -172.8032) -> (-410.9311, -163.6366)
  line L863 (-407.9311, -165.4723) -> (-407.9311, -156.3057)
  line L864 (-410.9311, -154.4699) -> (-410.9311, -159.0532)
  line L865 (-410.9311, -154.4699) -> (-410.9311, -149.8866)
  line L866 (-407.9311, -142.0103) -> (-407.9311, -151.177)
  line L867 (-410.9311, -136.1366) -> (-410.9311, -145.3032)
  line L868 (-406.0285, -172.8032) -> (-406.0285, -163.6366)
  line L869 (-403.0285, -165.4723) -> (-403.0285, -156.3057)
  line L870 (-406.0285, -154.4699) -> (-406.0285, -159.0532)
  line L871 (-406.0285, -154.4699) -> (-406.0285, -149.8866)
  line L872 (-403.0285, -142.0103) -> (-403.0285, -151.177)
  line L873 (-406.0285, -136.1366) -> (-406.0285, -145.3032)
  line L874 (-401.126, -172.8032) -> (-401.126, -163.6366)
  line L875 (-398.126, -165.4723) -> (-398.126, -156.3057)
  line L876 (-401.126, -154.4699) -> (-401.126, -159.0532)
  line L877 (-401.126, -154.4699) -> (-401.126, -149.8866)
  line L878 (-398.126, -142.0103) -> (-398.126, -151.177)
  line L879 (-401.126, -136.1366) -> (-401.126, -145.3032)
  line L880 (-396.2235, -172.8032) -> (-396.2235, -163.6366)
  line L881 (-393.2235, -165.4723) -> (-393.2235, -156.3057)
  line L882 (-396.2235, -154.4699) -> (-396.2235, -159.0532)
  line L883 (-396.2235, -154.4699) -> (-396.2235, -149.8866)
  line L884 (-393.2235, -142.0103) -> (-393.2235, -151.177)
  line L885 (-396.2235, -136.1366) -> (-396.2235, -145.3032)
  line L886 (-391.321, -172.8032) -> (-391.321, -163.6366)
  line L887 (-388.321, -165.4723) -> (-388.321, -156.3057)
  line L888 (-391.321, -154.4699) -> (-391.321, -159.0532)
  line L889 (-391.321, -154.4699) -> (-391.321, -149.8866)
  line L890 (-388.321, -142.0103) -> (-388.321, -151.177)
  line L891 (-391.321, -136.1366) -> (-391.321, -145.3032)
  line L892 (-386.4184, -172.8032) -> (-386.4184, -163.6366)
  line L893 (-383.4184, -165.4723) -> (-383.4184, -156.3057)
  line L894 (-386.4184, -154.4699) -> (-386.4184, -159.0532)
  line L895 (-386.4184, -154.4699) -> (-386.4184, -149.8866)
  line L896 (-383.4184, -142.0103) -> (-383.4184, -151.177)
  line L897 (-386.4184, -136.1366) -> (-386.4184, -145.3032)
  line L898 (-381.5159, -172.8032) -> (-381.5159, -163.6366)
  line L899 (-378.5159, -165.4723) -> (-378.5159, -156.3057)
  line L900 (-381.5159, -154.4699) -> (-381.5159, -159.0532)
  line L901 (-381.5159, -154.4699) -> (-381.5159, -149.8866)
  line L902 (-378.5159, -142.0103) -> (-378.5159, -151.177)
  line L903 (-381.5159, -136.1366) -> (-381.5159, -145.3032)
  line L904 (-376.6134, -172.8032) -> (-376.6134, -163.6366)
  line L905 (-373.6134, -165.4723) -> (-373.6134, -156.3057)
  line L906 (-376.6134, -154.4699) -> (-376.6134, -159.0532)
  line L907 (-376.6134, -154.4699) -> (-376.6134, -149.8866)
  line L908 (-373.6134, -142.0103) -> (-373.6134, -151.177)
  line L909 (-376.6134, -136.1366) -> (-376.6134, -145.3032)
  line L910 (-371.7109, -172.8032) -> (-371.7109, -163.6366)
  line L911 (-368.7109, -165.4723) -> (-368.7109, -156.3057)
  line L912 (-371.7109, -154.4699) -> (-371.7109, -159.0532)
  line L913 (-371.7109, -154.4699) -> (-371.7109, -149.8866)
  line L914 (-368.7109, -142.0103) -> (-368.7109, -151.177)
  line L915 (-371.7109, -136.1366) -> (-371.7109, -145.3032)
  circle A10 centre (-490.3726, -246.4167) radius 7.5
  circle A11 centre (-540.3726, -246.4167) radius 7.5
  circle A12 centre (-565.3726, -246.4167) radius 7.5
  circle A13 centre (-515.3726, -246.4167) radius 7.5
  line L916 (-582.5912, -193.3936) -> (-472.5912, -193.3936)
  line L917 (-472.5912, -193.3936) -> (-472.5912, -263.3936)
  line L918 (-472.5912, -263.3936) -> (-582.5912, -263.3936)
  line L919 (-582.5912, -263.3936) -> (-582.5912, -193.3936)
  line L920 (-565.3726, -208.3337) -> (-540.3726, -208.3337)
  line L921 (-540.3726, -208.3337) -> (-540.3726, -216.3337)
  line L922 (-540.3726, -216.3337) -> (-565.3726, -216.3337)
  line L923 (-565.3726, -216.3337) -> (-565.3726, -208.3337)
  line L924 (-490.3726, -208.4498) -> (-515.3726, -208.4498)
  line L925 (-515.3726, -208.4498) -> (-515.3726, -216.4498)
  line L926 (-515.3726, -216.4498) -> (-490.3726, -216.4498)
  line L927 (-490.3726, -216.4498) -> (-490.3726, -208.4498)
  circle A14 centre (-490.3726, -258.3944) radius 1.5
  circle A15 centre (-517.6226, -258.4373) radius 1.5
  circle A16 centre (-540.3726, -258.413) radius 1.5
  circle A17 centre (-563.1226, -258.413) radius 1.5
  circle A18 centre (-513.1226, -258.4373) radius 1.5
  circle A19 centre (-544.8726, -258.413) radius 1.5
  circle A20 centre (-535.8726, -258.413) radius 1.5
  circle A21 centre (-558.6226, -258.413) radius 1.5
  circle A22 centre (-572.1226, -258.413) radius 1.5
  circle A23 centre (-567.6226, -258.413) radius 1.5
  line L928 (-366.8083, -172.8032) -> (-366.8083, -163.6366)
  line L929 (-363.8083, -165.4723) -> (-363.8083, -156.3057)
  line L930 (-366.8083, -154.4699) -> (-366.8083, -159.0532)
  line L931 (-366.8083, -154.4699) -> (-366.8083, -149.8866)
  line L932 (-363.8083, -142.0103) -> (-363.8083, -151.177)
  line L933 (-366.8083, -136.1366) -> (-366.8083, -145.3032)
  line L934 (-361.9058, -172.8032) -> (-361.9058, -163.6366)
  line L935 (-358.9058, -165.4723) -> (-358.9058, -156.3057)
  line L936 (-361.9058, -154.4699) -> (-361.9058, -159.0532)
  line L937 (-361.9058, -154.4699) -> (-361.9058, -149.8866)
  line L938 (-358.9058, -142.0103) -> (-358.9058, -151.177)
  line L939 (-361.9058, -136.1366) -> (-361.9058, -145.3032)
  line L940 (-357.0033, -172.8032) -> (-357.0033, -163.6366)
  line L941 (-354.0033, -165.4723) -> (-354.0033, -156.3057)
  line L942 (-357.0033, -154.4699) -> (-357.0033, -159.0532)
  line L943 (-357.0033, -154.4699) -> (-357.0033, -149.8866)
  line L944 (-354.0033, -142.0103) -> (-354.0033, -151.177)
  line L945 (-357.0033, -136.1366) -> (-357.0033, -145.3032)
  line L946 (-352.1007, -172.8032) -> (-352.1007, -163.6366)
  line L947 (-349.1007, -165.4723) -> (-349.1007, -156.3057)
  line L948 (-352.1007, -154.4699) -> (-352.1007, -159.0532)
  line L949 (-352.1007, -154.4699) -> (-352.1007, -149.8866)
  line L950 (-349.1007, -142.0103) -> (-349.1007, -151.177)
  line L951 (-352.1007, -136.1366) -> (-352.1007, -145.3032)
  line L952 (-744.4974, -101.8126) -> (-594.4974, -101.8126)
  line L953 (-594.4974, -101.8126) -> (-594.4974, -262.8126)
  line L954 (-594.4974, -262.8126) -> (-744.4974, -262.8126)
  line L955 (-744.4974, -262.8126) -> (-744.4974, -101.8126)
  line L956 (-723.5897, -101.8126) -> (-613.9057, -101.8126)
  line L957 (-613.9057, -101.8126) -> (-613.9057, -226.5227)
  line L958 (-628.9057, -241.5227) -> (-708.5897, -241.5227)
  circle A24 centre (-723.5897, -241.5227) radius 7.5
  circle A25 centre (-613.9057, -241.5227) radius 7.5
  circle A26 centre (-723.5897, -142.0206) radius 7.5
  line L959 (-723.5897, -226.5227) -> (-723.5897, -157.0206)
  line L960 (-723.5897, -127.0206) -> (-723.5897, -101.8126)
  circle A27 centre (-668.6247, -182.3126) radius 37.5
  arc A28 (-708.5897, -241.5227) -> (-723.5897, -226.5227) centre (-723.5897, -241.5227) ccw
  arc A29 (-613.9057, -226.5227) -> (-628.9057, -241.5227) centre (-613.9057, -241.5227) ccw
  arc A30 (-723.5897, -157.0206) -> (-723.5897, -127.0206) centre (-723.5897, -142.0206) ccw
  line L961 (-646.8057, -111.5227) -> (-620.8595, -111.5227)
  line L962 (-618.7595, -113.6227) -> (-618.7595, -117.6991)
  line L963 (-620.8595, -119.7991) -> (-646.8057, -119.7991)
  line L964 (-648.9057, -117.6991) -> (-648.9057, -113.6227)
  arc A31 (-646.8057, -111.5227) -> (-648.9057, -113.6227) centre (-646.8057, -113.6227) ccw
  arc A32 (-648.9057, -117.6991) -> (-646.8057, -119.7991) centre (-646.8057, -117.6991) ccw
  arc A33 (-620.8595, -119.7991) -> (-618.7595, -117.6991) centre (-620.8595, -117.6991) ccw
  arc A34 (-618.7595, -113.6227) -> (-620.8595, -111.5227) centre (-620.8595, -113.6227) ccw
  arc A35 (-658.9057, -241.5227) -> (-678.9057, -241.5227) centre (-668.9057, -249.2998) ccw
  line L965 (-583.2827, -153.6352) -> (-478.2827, -153.6352)
  line L966 (-478.2827, -153.6352) -> (-478.2827, -175.6352)
  line L967 (-478.2827, -175.6352) -> (-583.2827, -175.6352)
  line L968 (-583.2827, -175.6352) -> (-583.2827, -153.6352)
  line L969 (-478.2827, -155.6352) -> (-478.2827, -157.6352)
  line L970 (-583.2827, -157.6352) -> (-583.2827, -155.6352)
  line L971 (-583.2827, -155.6352) -> (-573.2827, -155.6352)
  line L972 (-563.2827, -155.6352) -> (-553.2827, -155.6352)
  line L973 (-543.2827, -155.6352) -> (-533.2827, -155.6352)
  line L974 (-523.2827, -155.6352) -> (-513.2827, -155.6352)
  line L975 (-503.2827, -155.6352) -> (-493.2827, -155.6352)
  line L976 (-483.2827, -155.6352) -> (-478.2827, -155.6352)
  line L977 (-478.2827, -157.6352) -> (-488.2827, -157.6352)
  line L978 (-498.2827, -157.6352) -> (-508.2827, -157.6352)
  line L979 (-518.2827, -157.6352) -> (-528.2827, -157.6352)
  line L980 (-538.2827, -157.6352) -> (-548.2827, -157.6352)
  line L981 (-558.2827, -157.6352) -> (-568.2827, -157.6352)
  line L982 (-578.2827, -155.6352) -> (-573.2827, -155.6352)
  line L983 (-583.2827, -157.6352) -> (-578.2827, -157.6352)
  line L984 (-483.2827, -159.6352) -> (-478.2827, -159.6352)
  line L985 (-478.2827, -161.6352) -> (-488.2827, -161.6352)
  line L986 (-503.2827, -159.6352) -> (-493.2827, -159.6352)
  line L987 (-498.2827, -161.6352) -> (-508.2827, -161.6352)
  line L988 (-523.2827, -159.6352) -> (-513.2827, -159.6352)
  line L989 (-518.2827, -161.6352) -> (-528.2827, -161.6352)
  line L990 (-543.2827, -159.6352) -> (-533.2827, -159.6352)
  line L991 (-538.2827, -161.6352) -> (-548.2827, -161.6352)
  line L992 (-563.2827, -159.6352) -> (-553.2827, -159.6352)
  line L993 (-558.2827, -161.6352) -> (-568.2827, -161.6352)
  line L994 (-583.2827, -159.6352) -> (-573.2827, -159.6352)
  line L995 (-583.2827, -161.6352) -> (-578.2827, -161.6352)
  line L996 (-483.2827, -163.6352) -> (-478.2827, -163.6352)
  line L997 (-478.2827, -165.6352) -> (-488.2827, -165.6352)
  line L998 (-503.2827, -163.6352) -> (-493.2827, -163.6352)
  line L999 (-498.2827, -165.6352) -> (-508.2827, -165.6352)
  line L1000 (-523.2827, -163.6352) -> (-513.2827, -163.6352)
  line L1001 (-518.2827, -165.6352) -> (-528.2827, -165.6352)
  line L1002 (-543.2827, -163.6352) -> (-533.2827, -163.6352)
  line L1003 (-538.2827, -165.6352) -> (-548.2827, -165.6352)
  line L1004 (-563.2827, -163.6352) -> (-553.2827, -163.6352)
  line L1005 (-558.2827, -165.6352) -> (-568.2827, -165.6352)
  line L1006 (-583.2827, -163.6352) -> (-573.2827, -163.6352)
  line L1007 (-583.2827, -165.6352) -> (-578.2827, -165.6352)
  line L1008 (-483.2827, -167.6352) -> (-478.2827, -167.6352)
  line L1009 (-478.2827, -169.6352) -> (-488.2827, -169.6352)
  line L1010 (-503.2827, -167.6352) -> (-493.2827, -167.6352)
  line L1011 (-498.2827, -169.6352) -> (-508.2827, -169.6352)
  line L1012 (-523.2827, -167.6352) -> (-513.2827, -167.6352)
  line L1013 (-518.2827, -169.6352) -> (-528.2827, -169.6352)
  line L1014 (-543.2827, -167.6352) -> (-533.2827, -167.6352)
  line L1015 (-538.2827, -169.6352) -> (-548.2827, -169.6352)
  line L1016 (-563.2827, -167.6352) -> (-553.2827, -167.6352)
  line L1017 (-558.2827, -169.6352) -> (-568.2827, -169.6352)
  line L1018 (-583.2827, -167.6352) -> (-573.2827, -167.6352)
  line L1019 (-583.2827, -169.6352) -> (-578.2827, -169.6352)
  line L1020 (-483.2827, -171.6352) -> (-478.2827, -171.6352)
  line L1021 (-478.2827, -173.6352) -> (-488.2827, -173.6352)
  line L1022 (-503.2827, -171.6352) -> (-493.2827, -171.6352)
  line L1023 (-498.2827, -173.6352) -> (-508.2827, -173.6352)
  line L1024 (-523.2827, -171.6352) -> (-513.2827, -171.6352)
  line L1025 (-518.2827, -173.6352) -> (-528.2827, -173.6352)
  line L1026 (-543.2827, -171.6352) -> (-533.2827, -171.6352)
  line L1027 (-538.2827, -173.6352) -> (-548.2827, -173.6352)
  line L1028 (-563.2827, -171.6352) -> (-553.2827, -171.6352)
  line L1029 (-558.2827, -173.6352) -> (-568.2827, -173.6352)
  line L1030 (-583.2827, -171.6352) -> (-573.2827, -171.6352)
  line L1031 (-583.2827, -173.6352) -> (-578.2827, -173.6352)
  line L1032 (-655.8826, -103.5305) -> (-725.8826, -103.5305) construction
  line L1033 (-725.8826, -103.5305) -> (-725.8826, -73.5305) construction
  line L1034 (-725.8826, -73.5305) -> (-655.8826, -73.5305) construction
  line L1035 (-655.8826, -73.5305) -> (-655.8826, -103.5305) construction
  line L1036 (-499.0124, -156.4742) -> (-569.0124, -156.4742) construction
  line L1037 (-569.0124, -156.4742) -> (-569.0124, -126.4742) construction
  line L1038 (-569.0124, -126.4742) -> (-499.0124, -126.4742) construction
  line L1039 (-499.0124, -126.4742) -> (-499.0124, -156.4742) construction
  line L1040 (-516.0067, -312.6909) -> (-586.0067, -312.6909) construction
  line L1041 (-586.0067, -312.6909) -> (-586.0067, -282.6909) construction
  line L1042 (-586.0067, -282.6909) -> (-516.0067, -282.6909) construction
  line L1043 (-516.0067, -282.6909) -> (-516.0067, -312.6909) construction
  line L1044 (-210.1102, -313.3445) -> (-280.1102, -313.3445) construction
  line L1045 (-280.1102, -313.3445) -> (-280.1102, -283.3445) construction
  line L1046 (-280.1102, -283.3445) -> (-210.1102, -283.3445) construction
  line L1047 (-210.1102, -283.3445) -> (-210.1102, -313.3445) construction
  line L1048 (-368.9408, -312.0372) -> (-438.9408, -312.0372) construction
  line L1049 (-438.9408, -312.0372) -> (-438.9408, -282.0372) construction
  line L1050 (-438.9408, -282.0372) -> (-368.9408, -282.0372) construction
  line L1051 (-368.9408, -282.0372) -> (-368.9408, -312.0372) construction
  line L1052 (-363.0582, -134.251) -> (-433.0582, -134.251) construction
  line L1053 (-433.0582, -134.251) -> (-433.0582, -104.251) construction
  line L1054 (-433.0582, -104.251) -> (-363.0582, -104.251) construction
  line L1055 (-363.0582, -104.251) -> (-363.0582, -134.251) construction
  line L1056 (-105.5884, -127.1918) -> (-175.5884, -127.1918) construction
  line L1057 (-175.5884, -127.1918) -> (-175.5884, -97.1918) construction
  line L1058 (-175.5884, -97.1918) -> (-105.5884, -97.1918) construction
  line L1059 (-105.5884, -97.1918) -> (-105.5884, -127.1918) construction
  line L1060 (37.6145, -304.8473) -> (-32.3855, -304.8473) construction
  line L1061 (-32.3855, -304.8473) -> (-32.3855, -274.8473) construction
  line L1062 (-32.3855, -274.8473) -> (37.6145, -274.8473) construction
  line L1063 (37.6145, -274.8473) -> (37.6145, -304.8473) construction
  line L1064 (266.3836, -304.8473) -> (196.3836, -304.8473) construction
  line L1065 (196.3836, -304.8473) -> (196.3836, -274.8473) construction
  line L1066 (196.3836, -274.8473) -> (266.3836, -274.8473) construction
  line L1067 (266.3836, -274.8473) -> (266.3836, -304.8473) construction
  line L1068 (436.6546, -300.2702) -> (366.6546, -300.2702) construction
  line L1069 (366.6546, -300.2702) -> (366.6546, -270.2702) construction
  line L1070 (366.6546, -270.2702) -> (436.6546, -270.2702) construction
  line L1071 (436.6546, -270.2702) -> (436.6546, -300.2702) construction
  point P0 (-486.0714, -195.0863)
  point P1 (-552.0714, -195.0863)
  dimension "d124" = 55
  dimension "d127" = 330
  dimension "d128" = 0
  dimension "d129" = 945.4906
  dimension "d131" = 120.75
  dimension "d132" = 36.6667
  dimension "d133" = 3
  dimension "d134" = 9.1667
  dimension "d135" = 9.1667
  dimension "d136" = 9.1667
  dimension "d137" = 9.1667
  dimension "d138" = 4.5833
  dimension "d139" = 4.5833
  dimension "d145" = 93.148
  dimension "d146" = 0
  dimension "d147" = 8
  dimension "d148" = 8
  dimension "d149" = 3
  dimension "d150" = 3
  dimension "d151" = 3
  dimension "d152" = 3
  dimension "d168" = 150
  dimension "d169" = 161
  dimension "d170" = 15
  dimension "d171" = 15
  dimension "d172" = 15
  dimension "d173" = 75
  dimension "d174" = 15
  dimension "d176" = 15
  dimension "d178" = 15
  dimension "d180" = 2.1
  dimension "d181" = 109.6841
  dimension "d182" = 105
  dimension "d183" = 22
  dimension "d186" = 4
  dimension "d187" = 0
  dimension "d188" = 10
  dimension "d189" = 10
  dimension "d190" = 10
  dimension "d191" = 10
  dimension "d192" = 10
  dimension "d193" = 10
  dimension "d194" = 10
  dimension "d195" = 10
  dimension "d196" = 10
  dimension "d197" = 10
  constraint horizontal L780
  constraint horizontal L786
  constraint vertical L787
  constraint horizontal L788
  constraint vertical L789
  constraint horizontal L790
  constraint vertical L791
  constraint horizontal L792
  constraint vertical L793
  constraint horizontal L794
  constraint vertical L795
  constraint horizontal L796
  constraint vertical L797
  constraint horizontal L798
  constraint vertical L799
  constraint horizontal L800
  constraint vertical L801
  constraint perpendicular L797 L802
  constraint perpendicular L796 L803
  constraint perpendicular L797 L805
  constraint perpendicular L802 L807
  constraint perpendicular L800 L808
  constraint perpendicular L650 L810
  constraint perpendicular L810 L812
  constraint perpendicular L808 L813
  constraint horizontal L814
  constraint vertical L815
  constraint horizontal L816
  constraint vertical L817
  constraint horizontal L818
  constraint horizontal L819
  constraint coincident L816 L819.start
  constraint coincident L814 L818.start
  constraint perpendicular L819 L820
  constraint perpendicular L818 L821
  constraint horizontal L916
  constraint horizontal L918
  constraint vertical L919
  constraint horizontal L920
  constraint vertical L921
  constraint horizontal L922
  constraint vertical L923
  constraint horizontal L924
  constraint vertical L925
  constraint horizontal L926
  constraint vertical L927
  constraint horizontal L952
  constraint vertical L953
  constraint horizontal L954
  constraint vertical L955
  constraint horizontal L956
  constraint vertical L957
  constraint horizontal L958
  constraint vertical L959
  constraint coincident L952 L956.start
  constraint coincident A26.centre L959
  constraint collinear L959 L960
  constraint coincident A24.centre A28.centre
  constraint coincident A25.centre A29.centre
  constraint coincident A26.centre A30.centre
  constraint horizontal L961
  constraint vertical L962
  constraint horizontal L963
  constraint vertical L964
  constraint tangent L961 A31
  constraint tangent L964 A31
  constraint tangent L963 A32
  constraint tangent L964 A32
  constraint equal A31 A32
  constraint tangent L962 A33
  constraint tangent L963 A33
  constraint equal A31 A33
  constraint tangent L961 A34
  constraint tangent L962 A34
  constraint equal A31 A34
  constraint coincident L958 A35.start
  constraint coincident L958 A35.end
  constraint horizontal L965
  constraint vertical L966
  constraint horizontal L967
  constraint vertical L968
  constraint vertical L969
  constraint vertical L970
  constraint coincident L966 L969.end
  constraint coincident L968 L970.end
  constraint perpendicular L969 L978
  constraint midpoint L971 L982.start
  constraint perpendicular L968 L983
  measures "d124" distance of L780.start L780.end
  measures "d129" distance of L748 L793
  measures "d131" distance of L814.start L814.end
  measures "d132" distance of L814.start L816.end
  measures "d133" distance of L818.start L818.end
  measures "d134" distance of L819.end L820.end
  measures "d135" distance of L818.start L821.end
  measures "d136" distance of L822.start L822.end
  measures "d137" distance of L823.start L823.end
  measures "d138" distance of L824.start L824.end
  measures "d139" distance of L824.start L825.end
  measures "d147" distance of L920.start L922.end
  measures "d148" distance of L924.start L926.end
  measures "d149" diameter of A14
  measures "d150" diameter of A15
  measures "d151" diameter of A16
  measures "d152" diameter of A17
  measures "d168" distance of L952.start L952.end
  measures "d169" distance of L952.start L954.end
  measures "d170" diameter of A24
  measures "d171" diameter of A25
  measures "d172" diameter of A26
  measures "d173" diameter of A27
  measures "d174" radius of A28
  measures "d176" radius of A29
  measures "d178" radius of A30
  measures "d180" radius of A31
  measures "d181" distance of L957 L960
  measures "d182" distance of L965.start L965.end
  measures "d183" distance of L965.end L966.end